Autodesk Inventor part; units mm, degrees
(part 3 of 3)
  line L956 (-2.853, -22.3763) -> (-1.8481, -26.5214)
  line L957 (-1.8481, -26.5214) -> (-0.8514, -22.3763)
  line L958 (-0.8514, -22.3763) -> (-0.1747, -22.3763)
  line L959 (-0.1747, -22.3763) -> (0.8302, -26.57)
  line L960 (0.8302, -26.57) -> (1.831, -22.3763)
  line L961 (1.831, -22.3763) -> (2.4833, -22.3763)
  spline S382 degree 2 poles (4.4728, -27.4655) (3.9298, -27.4655) (3.1681, -27.2386) (2.8318, -27.0765) knots 0 0 0 1 2 2 2
  line L962 (2.8318, -27.0765) -> (2.8318, -26.2418)
  line L963 (2.8318, -26.2418) -> (2.8804, -26.2418)
  spline S383 degree 2 poles (2.8804, -26.2418) (3.2086, -26.5497) (4.0392, -26.8901) (4.4242, -26.8901) knots 0 0 0 1 2 2 2
  spline S384 degree 2 poles (4.4242, -26.8901) (4.9752, -26.8901) (5.5384, -26.4322) (5.5384, -26.0554) knots 0 0 0 1 2 2 2
  spline S385 degree 2 poles (5.5384, -26.0554) (5.5384, -25.7556) (5.2426, -25.3828) (4.9225, -25.2896) knots 0 0 0 1 2 2 2
  spline S386 degree 2 poles (4.9225, -25.2896) (4.6916, -25.2248) (4.3067, -25.1356) (4.019, -25.0627) knots 0 0 0 1 2 2 2
  spline S387 degree 2 poles (4.019, -25.0627) (3.7597, -24.9938) (3.3504, -24.7872) (3.1924, -24.6211) knots 0 0 0 1 2 2 2
  spline S388 degree 2 poles (3.1924, -24.6211) (3.0384, -24.4549) (2.8683, -24.0092) (2.8683, -23.7175) knots 0 0 0 1 2 2 2
  spline S389 degree 2 poles (2.8683, -23.7175) (2.8683, -23.1097) (3.8164, -22.2872) (4.5498, -22.2872) knots 0 0 0 1 2 2 2
  spline S390 degree 2 poles (4.5498, -22.2872) (4.9712, -22.2872) (5.7167, -22.4533) (6.0368, -22.6113) knots 0 0 0 1 2 2 2
  line L964 (6.0368, -22.6113) -> (6.0368, -23.4055)
  line L965 (6.0368, -23.4055) -> (5.9882, -23.4055)
  spline S391 degree 2 poles (5.9882, -23.4055) (5.7491, -23.1867) (5.0036, -22.8625) (4.5943, -22.8625) knots 0 0 0 1 2 2 2
  spline S392 degree 2 poles (4.5943, -22.8625) (4.1324, -22.8625) (3.5611, -23.2961) (3.5611, -23.6486) knots 0 0 0 1 2 2 2
  spline S393 degree 2 poles (3.5611, -23.6486) (3.5611, -23.9646) (3.8974, -24.3415) (4.2135, -24.4266) knots 0 0 0 1 2 2 2
  spline S394 degree 2 poles (4.2135, -24.4266) (4.4242, -24.4833) (5.036, -24.6292) (5.2386, -24.6899) knots 0 0 0 1 2 2 2
  spline S395 degree 2 poles (5.2386, -24.6899) (5.7532, -24.848) (6.2313, -25.4841) (6.2313, -25.9501) knots 0 0 0 1 2 2 2
  spline S396 degree 2 poles (6.2313, -25.9501) (6.2313, -26.2458) (5.9922, -26.8131) (5.7775, -27.0117) knots 0 0 0 1 2 2 2
  spline S397 degree 2 poles (5.7775, -27.0117) (5.5384, -27.2305) (4.9307, -27.4655) (4.4728, -27.4655) knots 0 0 0 1 2 2 2
  line L966 (10.5546, -27.3763) -> (9.6916, -27.3763)
  line L967 (9.6916, -27.3763) -> (7.8642, -25.0505)
  line L968 (7.8642, -25.0505) -> (7.5725, -25.3787)
  line L969 (7.5725, -25.3787) -> (7.5725, -27.3763)
  line L970 (7.5725, -27.3763) -> (6.908, -27.3763)
  line L971 (6.908, -27.3763) -> (6.908, -22.3763)
  line L972 (6.908, -22.3763) -> (7.5725, -22.3763)
  line L973 (7.5725, -22.3763) -> (7.5725, -24.6737)
  line L974 (7.5725, -24.6737) -> (9.6227, -22.3763)
  line L975 (9.6227, -22.3763) -> (10.4331, -22.3763)
  line L976 (10.4331, -22.3763) -> (8.3626, -24.6089)
  line L977 (8.3626, -24.6089) -> (10.5546, -27.3763)
  line L978 (12.694, -27.3763) -> (10.7572, -27.3763)
  line L979 (10.7572, -27.3763) -> (10.7572, -26.8658)
  line L980 (10.7572, -26.8658) -> (11.3934, -26.8658)
  line L981 (11.3934, -26.8658) -> (11.3934, -22.8869)
  line L982 (11.3934, -22.8869) -> (10.7572, -22.8869)
  line L983 (10.7572, -22.8869) -> (10.7572, -22.3763)
  line L984 (10.7572, -22.3763) -> (12.694, -22.3763)
  line L985 (12.694, -22.3763) -> (12.694, -22.8869)
  line L986 (12.694, -22.8869) -> (12.0579, -22.8869)
  line L987 (12.0579, -22.8869) -> (12.0579, -26.8658)
  line L988 (12.0579, -26.8658) -> (12.694, -26.8658)
  line L989 (12.694, -26.8658) -> (12.694, -27.3763)
  line L990 (13.5166, -27.3763) -> (13.5166, -22.3763)
  line L991 (13.5166, -22.3763) -> (16.6446, -22.3763)
  line L992 (16.6446, -22.3763) -> (16.6446, -22.9679)
  line L993 (16.6446, -22.9679) -> (14.1811, -22.9679)
  line L994 (14.1811, -22.9679) -> (14.1811, -24.3374)
  line L995 (14.1811, -24.3374) -> (16.4785, -24.3374)
  line L996 (16.4785, -24.3374) -> (16.4785, -24.929)
  line L997 (16.4785, -24.929) -> (14.1811, -24.929)
  line L998 (14.1811, -24.929) -> (14.1811, -26.7847)
  line L999 (14.1811, -26.7847) -> (16.6446, -26.7847)
  line L1000 (16.6446, -26.7847) -> (16.6446, -27.3763)
  line L1001 (16.6446, -27.3763) -> (13.5166, -27.3763)
  spline S398 degree 2 poles (19.4687, -27.4736) (18.9379, -27.4736) (18.0587, -27.1494) (17.7426, -26.8212) knots 0 0 0 1 2 2 2
  spline S399 degree 2 poles (17.7426, -26.8212) (17.4266, -26.489) (17.0903, -25.5084) (17.0903, -24.8723) knots 0 0 0 1 2 2 2
  spline S400 degree 2 poles (17.0903, -24.8723) (17.0903, -24.2685) (17.4307, -23.3123) (17.7467, -22.9719) knots 0 0 0 1 2 2 2
  spline S401 degree 2 poles (17.7467, -22.9719) (18.0506, -22.6437) (18.942, -22.2872) (19.4728, -22.2872) knots 0 0 0 1 2 2 2
  spline S402 degree 2 poles (19.4728, -22.2872) (19.7281, -22.2872) (20.19, -22.3601) (20.4007, -22.4249) knots 0 0 0 1 2 2 2
  spline S403 degree 2 poles (20.4007, -22.4249) (20.5708, -22.4736) (20.9841, -22.6518) (21.1097, -22.7167) knots 0 0 0 1 2 2 2
  line L1002 (21.1097, -22.7167) -> (21.1097, -23.5189)
  line L1003 (21.1097, -23.5189) -> (21.053, -23.5189)
  spline S404 degree 2 poles (21.053, -23.5189) (20.9274, -23.4095) (20.664, -23.211) (20.4209, -23.0975) knots 0 0 0 1 2 2 2
  spline S405 degree 2 poles (20.4209, -23.0975) (20.2183, -22.9963) (19.6956, -22.8625) (19.3958, -22.8625) knots 0 0 0 1 2 2 2
  spline S406 degree 2 poles (19.3958, -22.8625) (18.6746, -22.8625) (17.7832, -23.9484) (17.7832, -24.852) knots 0 0 0 1 2 2 2
  spline S407 degree 2 poles (17.7832, -24.852) (17.7832, -25.3544) (18.0182, -26.1081) (18.241, -26.3674) knots 0 0 0 1 2 2 2
  spline S408 degree 2 poles (18.241, -26.3674) (18.4558, -26.6267) (19.0636, -26.8982) (19.4444, -26.8982) knots 0 0 0 1 2 2 2
  spline S409 degree 2 poles (19.4444, -26.8982) (19.724, -26.8982) (20.2832, -26.8172) (20.4736, -26.7361) knots 0 0 0 1 2 2 2
  line L1004 (20.4736, -26.7361) -> (20.4736, -25.4436)
  line L1005 (20.4736, -25.4436) -> (19.3148, -25.4436)
  line L1006 (19.3148, -25.4436) -> (19.3148, -24.8601)
  line L1007 (19.3148, -24.8601) -> (21.13, -24.8601)
  line L1008 (21.13, -24.8601) -> (21.13, -27.0441)
  spline S410 degree 2 poles (21.13, -27.0441) (21.0044, -27.1008) (20.5749, -27.275) (20.3926, -27.3277) knots 0 0 0 1 2 2 2
  spline S411 degree 2 poles (20.3926, -27.3277) (20.1454, -27.4006) (19.7483, -27.4736) (19.4687, -27.4736) knots 0 0 0 1 2 2 2
  spline S412 degree 2 poles (25.502, -22.9476) (25.7856, -23.2799) (26.1016, -24.2523) (26.1016, -24.8763) knots 0 0 0 1 2 2 2
  spline S413 degree 2 poles (26.1016, -24.8763) (26.1016, -25.4841) (25.7937, -26.4687) (25.502, -26.801) knots 0 0 0 1 2 2 2
  spline S414 degree 2 poles (25.502, -26.801) (25.194, -27.1494) (24.3796, -27.4817) (23.8893, -27.4817) knots 0 0 0 1 2 2 2
  spline S415 degree 2 poles (23.8893, -27.4817) (23.3828, -27.4817) (22.5725, -27.1373) (22.2767, -26.801) knots 0 0 0 1 2 2 2
  spline S416 degree 2 poles (22.2767, -26.801) (21.989, -26.4687) (21.6811, -25.4922) (21.6811, -24.8763) knots 0 0 0 1 2 2 2
  spline S417 degree 2 poles (21.6811, -24.8763) (21.6811, -24.2483) (21.9931, -23.292) (22.2807, -22.9476) knots 0 0 0 1 2 2 2
  spline S418 degree 2 poles (22.2807, -22.9476) (22.5725, -22.6154) (23.3869, -22.271) (23.8893, -22.271) knots 0 0 0 1 2 2 2
  spline S419 degree 2 poles (23.8893, -22.271) (24.3999, -22.271) (25.2183, -22.6275) (25.502, -22.9476) knots 0 0 0 1 2 2 2
  spline S420 degree 2 poles (25.4088, -24.8763) (25.4088, -24.382) (25.194, -23.6162) (24.9995, -23.365) knots 0 0 0 1 2 2 2
  spline S421 degree 2 poles (24.9995, -23.365) (24.801, -23.1057) (24.2418, -22.8463) (23.8934, -22.8463) knots 0 0 0 1 2 2 2
  spline S422 degree 2 poles (23.8934, -22.8463) (23.5328, -22.8463) (22.9898, -23.0975) (22.7832, -23.365) knots 0 0 0 1 2 2 2
  spline S423 degree 2 poles (22.7832, -23.365) (22.5846, -23.6202) (22.3739, -24.3901) (22.3739, -24.8763) knots 0 0 0 1 2 2 2
  spline S424 degree 2 poles (22.3739, -24.8763) (22.3739, -25.8609) (23.2005, -26.9063) (23.8934, -26.9063) knots 0 0 0 1 2 2 2
  spline S425 degree 2 poles (23.8934, -26.9063) (24.5862, -26.9063) (25.4088, -25.8609) (25.4088, -24.8763) knots 0 0 0 1 2 2 2
  point P0 (0, 0)
  constraints: 2 other
extrude "Wyciągnięcie proste2" add sketch "Szkic2" along normal blind 2
sketch "Szkic3" plane through (0, 2, 0) normal (0, 1, 0) x (1, 0, 0)
  line L0 (-45, 35) -> (45, 35)
  line L1 (45, 35) -> (45, -35)
  line L2 (45, -35) -> (-45, -35)
  line L3 (-45, -35) -> (-45, 35)
  line L4 (-45, 35) -> (45, -35) construction
  line L5 (45, 35) -> (-45, -35) construction
  circle A0 centre (-45, 35) radius 1.5
  circle A1 centre (45, 35) radius 1.5
  circle A2 centre (-45, -35) radius 1.5
  circle A3 centre (45, -35) radius 1.5
  point P0 (0, 0)
  dimension "d6" = 90
  dimension "d7" = 70
  dimension "d8" = 3
  dimension "d9" = 3
  dimension "d10" = 3
  dimension "d11" = 3
  constraints: 12 end point, 4 centre point, 4 coincident, 2 midpoint, 2 parallel, 1 horizontal, 1 perpendicular
  measures "d6" distance of L1.end L2.end
  measures "d7" distance of L0.end L1.end
  measures "d8" diameter of A0
  measures "d9" diameter of A1
  measures "d10" diameter of A2
  measures "d11" diameter of A3
extrude "Wyciągnięcie proste3" cut sketch "Szkic3" against normal blind 2 contours L3 A0 L0 | L0 A0 L3 | A1 L1 L0 | L0 L1 A1 | A2 L2 L3 | L3 L2 A2 | A3 L2 L1 | L1 L2 A3
fillet "Zaokrąglenie1" radius 4 4 edges at (-50, 1, 40) (50, 1, 40) (50, 1, -40) (-50, 1, -40)
chamfer "Faza1" distance 2 angle 45 4 edges at (-46.5, 2, -35) (-46.5, 2, 35) (43.5, 2, 35) (43.5, 2, -35)
